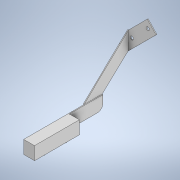
# Autodesk Inventor part: ventosas
Saved by Autodesk Inventor 2020 (Build 240168000, 168)
## iProperties
Created: 2022-11-11
Part Number: ventosas
Material: Genérico
Document SubType Name: Modeling
Designer: robin
Density: 1 g/cm^3
Appearance: Valor por defecto
Author: robin
Autodesk Inventor part; units mm, degrees
ref_plane "YZ Plane" through (0, 0, 0) normal (1, 0, 0) x (0, 1, 0)
ref_plane "XZ Plane" through (0, 0, 0) normal (0, 1, 0) x (-1, 0, 0)
ref_plane "XY Plane" through (0, 0, 0) normal (0, 0, 1) x (1, 0, 0)
sketch "Boceto1" plane through (0, 0, 0) normal (1, 0, 0) x (0, 1, 0)
  line L0 (0, 0) -> (-23.8, 0)
  line L1 (-23.8, 0) -> (-23.8, -81.8)
  line L2 (-23.8, -81.8) -> (0, -81.8)
  line L3 (0, -81.8) -> (0, 0)
  dimension "d0" = 23.8
  dimension "d1" = 81.8
  constraints: 8 end point, 2 parallel, 1 horizontal, 1 perpendicular
  measures "d0" distance of L2.end L1.end
  measures "d1" distance of L1.end L0.end
extrude "Extrusión1" add sketch "Boceto1" along normal blind 12.5
sketch "Boceto2" plane through (0, 0, 0) normal (-1, 0, 0) x (0, 0, 1)
  line L0 (0, 0) -> (-143, 0)
  line L1 (-143, 0) -> (-143, -13.8)
  line L2 (-133, -23.8) -> (0, -23.8)
  line L3 (0, -23.8) -> (0, 0)
  arc A0 (-143, -13.8) -> (-133, -23.8) centre (-133, -13.8) ccw
  point P0 (-143, -23.8)
  dimension "d4" = 143
  dimension "d5" = 10
  constraints: 8 end point, 2 parallel, 2 point on circle, 2 point on line, 2 tangent, 1 centre point, 1 horizontal, 1 perpendicular
  measures "d4" distance of L2.end point (-143, -23.8)
  measures "d5" radius of A0
extrude "Extrusión2" add sketch "Boceto2" along normal blind 1.55
sketch "Boceto3" plane through (-1.55, 0, 0) normal (-1, 0, 0) x (0, 0, 1)
  line L0 (-81.8, 0) -> (0, 0) projected
  line L1 (-143, 0) -> (-143, -13.8) projected
  line L2 (-143, 0) -> (-110.2, 0)
  line L3 (-81.8, 0) -> (-143, 0) projected
  line L4 (-143, 0) -> (-192.2511, 45.8653)
  arc A0 (-16.2, 0) -> (-135.0604, 90.653) centre (-110.2, 0) ccw
  line L5 (-176.372, 62.9165) -> (-110.2, 0)
  line L6 (-176.372, 62.9165) -> (-193.2664, 78.6495)
  line L7 (-192.2511, 45.8653) -> (-193.2664, 78.6495)
  dimension "d10" = 32.8
  dimension "d15" = 23.3
  dimension "d17" = 32.8
  constraints: 10 end point, 2 coincident, 2 point on circle, 2 point on line, 1 centre point
  measures "d10" distance of L1.start L2.end
  measures "d15" distance of L4.end L5.start
  measures "d17" distance of L6.end L4.end
extrude "Extrusión3" add sketch "Boceto3" along normal blind 1.55
sketch "Boceto6" plane through (-1.55, 45.8653, -192.2511) normal (0, -0.031, -0.9995) x (-1, 0, 0)
  circle A0 centre (1.55, 11.2988) radius 152.2645
  point P0 (-1.55, -51.7948)
  constraints: 1 centre point
extrude "Extrusión5" add sketch "Boceto6" against normal blind 1.55
sketch "Boceto7" plane through (-3.1, 57.2067, -191.0516) normal (0, 0.031, 0.9995) x (1, 0, 0)
  line L0 (1.55, -12.8346) -> (1.55, -58.6668) projected
  line L1 (1.55, -12.8346) -> (51.0475, 36.6629)
  line L2 (1.55, -12.8346) -> (71.55, -12.8346) construction
  line L3 (51.0475, 36.6629) -> (34.5719, 53.1385)
  line L4 (1.55, 5.2527) -> (1.55, 19.9654) projected
  line L5 (34.5719, 53.1385) -> (1.55, 19.9654)
  line L6 (1.55, 19.9654) -> (1.55, -12.8346)
  circle A0 centre (-14.9256, -12.8346) radius 218.7609
  point P0 (3.1, -63.0936)
  point P1 (1.55, 5.2527)
  dimension "d29" = 70
  dimension "d30" = 45
  dimension "d31" = 23.3
  constraints: 10 end point, 1 centre point, 1 equal length, 1 horizontal, 1 perpendicular
  measures "d29" distance of L0.start L1.end
  measures "d30" angle of L2 L1
  measures "d31" distance of L1.end L3.end
extrude "Extrusión6" cut sketch "Boceto7" against normal blind 1.55
sketch "Boceto8" plane through (-1.55, 44.3303, -192.2035) normal (0, -0.031, -0.9995) x (-0.7071, 0.7068, -0.0219)
  line L0 (0, 0) -> (0, 70) projected
  line L1 (0, 70) -> (23.3, 70) projected
  line L2 (24.2891, 22.0971) -> (1.096, -1.096) projected
  circle A0 centre (12.25, 20.808) radius 3
  circle A1 centre (12.25, 60.808) radius 3
  point P0 (-36.6345, -34.4425)
  dimension "d36" = 6
  dimension "d38" = 6
  constraints: 2 centre point
  measures "d36" diameter of A0
  measures "d38" diameter of A1
extrude "Extrusión7" cut sketch "Boceto8" against normal blind 1.55
sketch "Boceto11" plane through (12.5, 0, 0) normal (1, 0, 0) x (0, 0, -1)
  line L0 (0, -23.8) -> (0, 0) projected
  line L1 (133, -23.8) -> (81.8, -23.8) projected
  line L2 (0, 0) -> (81.8, 0)
  line L3 (81.8, 0) -> (81.8, -23.8)
  line L4 (81.8, -23.8) -> (0, -23.8)
  line L5 (0, -23.8) -> (0, 0)
  constraints: 8 end point, 2 parallel, 1 horizontal, 1 perpendicular
extrude "Extrusión9" add sketch "Boceto11" along normal blind 5.8
sketch "Boceto13" plane through (0, -23.8, -133) normal (0, -1, 0) x (1, 0, 0)
  line L0 (0, 51.2) -> (18.3, 51.2) projected
  circle A0 centre (9.15, 72.1) radius 6
  circle A1 centre (9.15, 112.1) radius 6
  point P0 (0, 133)
  dimension "d49" = 12
  dimension "d50" = 12
  constraints: 2 centre point
  measures "d49" diameter of A0
  measures "d50" diameter of A1
extrude "Extrusión10" add sketch "Boceto13" along normal blind 3.5
